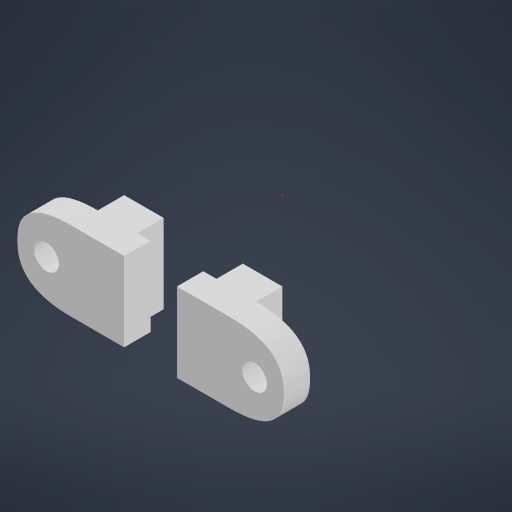
# Autodesk Inventor part: Connector_A
Saved by Autodesk Inventor 2024.1 (Build 281209000, 209)
## iProperties
Created: 2023-08-17
Part Number: Connector_A
Material: Generic
Document SubType Name: Modeling
Designer: Eleanor
Density: 1 g/cm^3
Appearance: Default
Author: Eleanor
Autodesk Inventor part; units mm, degrees
ref_plane "Work Plane6" through (0, 9.525, 0) normal (0, 1, 0) x (1, 0, 0)
sketch "Sketch6" plane through (0, 9.525, 0) normal (0, 1, 0) x (1, 0, 0)
  line L0 (9.525, -19.05) -> (-9.525, -19.05)
  line L1 (-9.525, -19.05) -> (-9.525, -25.4)
  line L2 (9.525, -25.4) -> (9.525, -19.05)
  line L3 (3.175, -22.225) -> (4.7625, -22.225)
  line L4 (-4.7625, 25.4) -> (4.7625, 25.4) projected
  line L5 (4.7625, 22.225) -> (4.7625, 25.4) projected
  line L6 (-4.7625, -22.225) -> (-3.175, -22.225)
  line L7 (-3.175, -22.225) -> (-3.175, -25.4)
  line L8 (-4.7625, -22.225) -> (-4.7625, -19.05)
  line L9 (4.7625, -22.225) -> (4.7625, -19.05)
  line L10 (3.175, -22.225) -> (3.175, -25.4)
  line L11 (-9.525, -25.4) -> (-3.175, -25.4)
  line L12 (3.175, -25.4) -> (9.525, -25.4)
  point P0 (0, 0)
  constraints: 22 end point, 7 perpendicular, 3 parallel, 3 point on line
extrude "Extrusion6" add sketch "Sketch6" against normal blind 9.525
ref_plane "Work Plane7" through (3.175, 9.525, 25.4) normal (0, 0, 1) x (1, 0, 0)
sketch "Sketch7" plane through (3.175, 9.525, 25.4) normal (0, 0, 1) x (1, 0, 0)
  circle A0 centre (9.35, -4.7625) radius 1.5
  line L0 (12.85, -5.0165) -> (12.85, -4.5085)
  line L1 (12.85, -4.5085) -> (12.85, 0) construction
  line L2 (12.85, 0) -> (6.35, 0) construction
  spline S0 degree 2 poles (12.85, -4.5085) (12.85, 0) (6.35, 0) knots 1 1 1 2 2 2
  line L3 (12.85, -5.0165) -> (12.85, -9.525) construction
  line L4 (12.85, -9.525) -> (6.35, -9.525) construction
  spline S1 degree 2 poles (12.85, -5.0165) (12.85, -9.525) (6.35, -9.525) knots 1 1 1 2 2 2
  line L5 (-3.175, -9.525) -> (-3.175, 0)
  line L6 (-7.9375, 0) -> (1.5875, 0) projected
  line L7 (6.35, 0) -> (6.35, -9.525) projected
  line L8 (6.35, -9.525) -> (6.35, 0)
  circle A1 centre (-15.7, -4.7625) radius 1.5
  line L9 (-19.2, -5.0165) -> (-19.2, -4.5085)
  line L10 (-19.2, -4.5085) -> (-19.2, 0) construction
  line L11 (-19.2, 0) -> (-12.7, 0) construction
  spline S2 degree 2 poles (-19.2, -4.5085) (-19.2, 0) (-12.7, 0) knots 1 1 1 2 2 2
  line L12 (-19.2, -5.0165) -> (-19.2, -9.525) construction
  line L13 (-19.2, -9.525) -> (-12.7, -9.525) construction
  spline S3 degree 2 poles (-19.2, -5.0165) (-19.2, -9.525) (-12.7, -9.525) knots 1 1 1 2 2 2
  line L14 (-12.7, 0) -> (-12.7, -9.525)
  line L15 (-12.7, -9.525) -> (-12.7, 0)
  point P0 (10.85, -4.7625)
  point P1 (-17.2, -4.7625)
  dimension "d25" = 3
  constraints: 12 end point, 8 symmetric about line, 3 vertical, 2 horizontal alignment, 2 point on line, 1 horizontal, 1 midpoint, 16 other
extrude "Extrusion7" add sketch "Sketch7" against normal blind 3.175
ref_plane "Work Plane5" through (-4.7625, 0, 3.175) normal (0, 0, 1) x (1, 0, 0)
ref_plane "Work Plane8" through (-9.525, 0, 22.225) normal (-1, 0, 0) x (0, 0, 1)
sketch "Sketch8" plane through (-9.525, 0, 22.225) normal (-1, 0, 0) x (0, 0, 1)
  point P0 (-22.225, 0)
body "Solid1"
